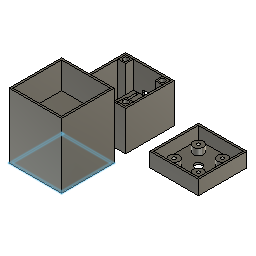
TeamsStatusLight (Autodesk Fusion 360 design; units mm, degrees)
Autodesk Fusion 360 part; units mm, degrees
sketch "Sketch1" plane through (0, 0, 0) normal (0, 0, 1) x (1, 0, 0)
  line L0 (1.4665, 38.7145) -> (39.4665, 38.7145)
  line L1 (39.4665, 38.7145) -> (39.4665, 0.7145)
  line L2 (39.4665, 0.7145) -> (1.4665, 0.7145)
  line L3 (1.4665, 0.7145) -> (1.4665, 38.7145)
  dimension "d4" = 38
  dimension "d5" = 38
  constraint horizontal L0
  constraint vertical L1
  constraint horizontal L2
  constraint vertical L3
  measures "d4" distance of L0.start L0.end
  measures "d5" distance of L0.start L2.end
extrude "Extrude1" add sketch "Sketch1" along normal blind 1.5 makes body 1
sketch "Sketch2" plane through (0, 0, 1.5) normal (0, 0, 1) x (-1, 0, 0)
  line L0 (-1.4665, -0.7145) -> (-39.4665, -0.7145)
  line L1 (-39.4665, -0.7145) -> (-39.4665, -38.7145)
  line L2 (-39.4665, -38.7145) -> (-1.4665, -38.7145)
  line L3 (-1.4665, -38.7145) -> (-1.4665, -0.7145)
  line L4 (-1.4665, -38.7145) -> (-2.9665, -38.7145)
  line L5 (-2.9665, -38.7145) -> (-2.9665, -37.2145)
  line L6 (-2.9665, -37.2145) -> (-37.9665, -37.2145)
  line L7 (-37.9665, -37.2145) -> (-37.9665, -2.2145)
  line L8 (-37.9665, -2.2145) -> (-2.9665, -2.2145)
  line L9 (-2.9665, -2.2145) -> (-2.9665, -37.2145)
  dimension "d8" = 1.5
  dimension "d9" = 1.5
  dimension "d10" = 35
  dimension "d11" = 35
  constraint coincident L2.end L3.start
  constraint perpendicular L3 L4
  constraint perpendicular L2 L5
  constraint horizontal L6
  constraint vertical L7
  constraint horizontal L8
  constraint vertical L9
  measures "d8" distance of L2.end L4.end
  measures "d9" distance of L4.end L5.end
  measures "d10" distance of L5.end L6.end
  measures "d11" distance of L5.end L8.end
extrude "Extrude2" add sketch "Sketch2" along normal blind 40 bodies 1
ref_plane "WorkPlane1" through (20.4665, 19.7145, 20.75) normal (0, 1, 0) x (-1, 0, 0)
ref_plane "WorkPlane2" through (20.4665, 19.7145, 20.75) normal (-1, 0, 0) x (0, -1, 0)
sketch "Sketch3" plane through (0, 38.7145, 0) normal (0, 1, 0) x (-1, 0, 0)
  line L0 (-39.4665, 0) -> (-1.4665, 0)
  line L1 (-1.4665, 0) -> (-1.4665, 41.5)
  line L2 (-1.4665, 41.5) -> (-39.4665, 41.5)
  line L3 (-39.4665, 41.5) -> (-39.4665, 0)
  line L4 (-20.4665, 0) -> (-20.4665, 1.5)
  line L5 (-20.4665, 1.5) -> (-20.4665, 12)
  line L6 (-16.9665, 13.75) -> (-23.9665, 13.75)
  line L7 (-24.9665, 12.75) -> (-24.9665, 11.25)
  line L8 (-23.9665, 10.25) -> (-16.9665, 10.25)
  line L9 (-15.9665, 11.25) -> (-15.9665, 12.75)
  line L10 (-15.9665, 13.75) -> (-24.9665, 10.25) construction
  line L11 (-24.9665, 13.75) -> (-15.9665, 10.25) construction
  arc A0 (-23.9665, 13.75) -> (-24.9665, 12.75) centre (-23.9665, 12.75) ccw
  arc A1 (-24.9665, 11.25) -> (-23.9665, 10.25) centre (-23.9665, 11.25) ccw
  arc A2 (-16.9665, 10.25) -> (-15.9665, 11.25) centre (-16.9665, 11.25) ccw
  arc A3 (-15.9665, 12.75) -> (-16.9665, 13.75) centre (-16.9665, 12.75) ccw
  point P0 (-20.4665, 12)
  dimension "d18" = 1.5
  dimension "d19" = 10.5
  dimension "d20" = 9
  dimension "d21" = 3.5
  dimension "d22" = 1
  constraint midpoint L0 L4.start
  constraint perpendicular L0 L4
  constraint parallel L4 L5
  constraint horizontal L6
  constraint perpendicular L6 L7
  constraint parallel L6 L8
  constraint parallel L7 L9
  constraint coincident L10 P0
  constraint coincident L11 P0
  constraint coincident P0 L5.end
  constraint coincident L11.start L6
  constraint coincident L11.start L7
  constraint tangent L6 A0
  constraint tangent L7 A0
  constraint coincident L10.end L7
  constraint coincident L10.end L8
  constraint tangent L7 A1
  constraint tangent L8 A1
  constraint equal A0 A1
  constraint coincident L11.end L9
  constraint coincident L11.end L8
  constraint tangent L9 A2
  constraint tangent L8 A2
  constraint equal A0 A2
  constraint coincident L10.start L9
  constraint coincident L10.start L6
  constraint tangent L9 A3
  constraint tangent L6 A3
  constraint equal A0 A3
  measures "d18" distance of L4.start L4.end
  measures "d19" distance of L4.end P0
  measures "d20" distance of L10.end L11.end
  measures "d21" distance of L11.start L10.end
  measures "d22" radius of A0
extrude "Extrude3" cut sketch "Sketch3" against normal blind 1.5 contours L6 L7 L8 L9 A0 A1 A2 A3 bodies 1
sketch "Sketch4" plane through (0, 0, 1.5) normal (0, 0, 1) x (-1, 0, 0)
  line L0 (-37.9665, -2.2145) -> (-37.9665, -37.2145)
  line L1 (-37.9665, -37.2145) -> (-2.9665, -37.2145)
  line L2 (-2.9665, -37.2145) -> (-2.9665, -2.2145)
  line L3 (-2.9665, -2.2145) -> (-37.9665, -2.2145)
  line L4 (-20.4665, -37.2145) -> (-20.4665, -25.4645)
  line L5 (-11.3165, -37.2145) -> (-29.6165, -37.2145)
  line L6 (-29.6165, -37.2145) -> (-29.6165, -13.7145)
  line L7 (-29.6165, -13.7145) -> (-11.3165, -13.7145)
  line L8 (-11.3165, -13.7145) -> (-11.3165, -37.2145)
  line L9 (-11.3165, -37.2145) -> (-29.6165, -13.7145) construction
  line L10 (-29.6165, -37.2145) -> (-11.3165, -13.7145) construction
  point P0 (-20.4665, -25.4645)
  dimension "d29" = 11.75
  dimension "d30" = 18.3
  dimension "d31" = 23.5
  constraint midpoint L1 L4.start
  constraint perpendicular L1 L4
  constraint horizontal L5
  constraint perpendicular L5 L6
  constraint parallel L5 L7
  constraint parallel L6 L8
  constraint coincident L9 P0
  constraint coincident L10 P0
  constraint coincident P0 L4.end
  measures "d29" distance of L4.start P0
  measures "d30" distance of L6.end L7.end
  measures "d31" distance of L5.end L6.end
extrude "Extrude4" add sketch "Sketch4" along normal blind 8.5 contours L1 L5 L6 L7 L8 bodies 1
sketch "Sketch5" plane through (0, 0, 10) normal (0, 0, 1) x (-1, 0, 0)
  line L0 (-11.3165, -13.7145) -> (-29.6165, -13.7145)
  line L1 (-29.6165, -13.7145) -> (-29.6165, -37.2145)
  line L2 (-29.6165, -37.2145) -> (-11.3165, -37.2145)
  line L3 (-11.3165, -37.2145) -> (-11.3165, -13.7145)
  line L4 (-29.6165, -13.7145) -> (-25.6165, -13.7145)
  line L5 (-25.6165, -13.7145) -> (-25.6165, -15.2145)
  point P0 (-22.9498, -15.2145)
  point P1 (-20.2831, -15.2145)
  point P2 (-17.6165, -15.2145)
  dimension "d34" = 4
  dimension "d35" = 1.5
  dimension "d38" = 8
  dimension "d39" = 0
  constraint coincident L0.end L1.start
  constraint perpendicular L1 L4
  constraint perpendicular L4 L5
  measures "d34" distance of L0.end L4.end
  measures "d35" distance of L4.end L5.end
hole "Hole1" at (25.6165, 15.2145, 10) at (22.9498, 15.2145, 10) at (20.2831, 15.2145, 10) at (17.6165, 15.2145, 10) direction (0, 0, -1) diameter 0.7 depth 7 tip angle 180 bodies 1
ref_plane "WorkPlane3" through (20.4665, 19.7145, 20.75) normal (0, 0, 1) x (1, 0, 0)
split "Split1" by plane through (20.4665, 19.7145, 20.75) normal (0, 0, 1) bodies 1 makes body 2 at (1.4665, 13.3812, 27.6667)
move_body "Move1" bodies 2 to x (1, 0, 0) y (0, 1, 0) z (0, 0, 1) at (57, 0, 0)
ref_plane "WorkPlane4" through (77.4665, 19.7145, 31.125) normal (1, 0, 0) x (0, 1, 0)
ref_plane "WorkPlane5" through (77.4665, 19.7145, 31.125) normal (0, 1, 0) x (-1, 0, 0)
sketch "Sketch6" plane through (0, 37.2145, 0) normal (0, -1, 0) x (1, 0, 0)
  line L0 (59.9665, 20.75) -> (94.9665, 20.75)
  line L1 (94.9665, 20.75) -> (94.9665, 41.5)
  line L2 (94.9665, 41.5) -> (59.9665, 41.5)
  line L3 (59.9665, 41.5) -> (59.9665, 20.75)
  line L4 (59.9665, 20.75) -> (94.9665, 20.75)
  line L5 (94.9665, 20.75) -> (94.9665, 22.25)
  line L6 (94.9665, 22.25) -> (59.9665, 22.25)
  line L7 (59.9665, 22.25) -> (59.9665, 20.75)
  dimension "d43" = 35
  dimension "d44" = 1.5
  constraint horizontal L4
  constraint vertical L5
  constraint horizontal L6
  constraint vertical L7
  constraint coincident L0.start L3.end
  measures "d43" distance of L0.start L0.end
  measures "d44" distance of L0.start L6.end
extrude "Extrude5" add sketch "Sketch6" along normal blind 35 contours L0 L1 L3 L4 L5 L6 L7 bodies 2
sketch "Sketch7" plane through (0, 0, 22.25) normal (0, 0, 1) x (-1, 0, 0)
  line L0 (-94.9665, -37.2145) -> (-59.9665, -37.2145)
  line L1 (-59.9665, -37.2145) -> (-59.9665, -2.2145)
  line L2 (-59.9665, -2.2145) -> (-94.9665, -2.2145)
  line L3 (-94.9665, -2.2145) -> (-94.9665, -37.2145)
  line L4 (-59.9665, -37.2145) -> (-67.9665, -37.2145)
  line L5 (-67.9665, -37.2145) -> (-67.9665, -29.2145)
  circle A0 centre (-67.9665, -29.2145) radius 4
  line L6 (-100.2665, -19.7145) -> (-54.6665, -19.7145)
  circle A1 centre (-67.9665, -10.2145) radius 4
  line L7 (-77.4665, 3.0855) -> (-77.4665, -42.5145)
  circle A2 centre (-86.9665, -29.2145) radius 4
  circle A3 centre (-86.9665, -10.2145) radius 4
  dimension "d47" = 8
  dimension "d50" = 8
  dimension "d51" = 8
  constraint coincident L0.end L1.start
  constraint perpendicular L1 L4
  constraint perpendicular L0 L5
  constraint coincident L5.end A0.centre
  constraint symmetric A0 L6 A1
  constraint symmetric A0 L7 A2
  constraint symmetric A1 L7 A3
  measures "d47" distance of L0.end L4.end
  measures "d50" distance of L4.end L5.end
  measures "d51" diameter of A0
extrude "Extrude6" add sketch "Sketch7" along normal blind 5 contours A0 | A1 | A2 | A3 bodies 2
hole "Hole3" at (67.9665, 29.2145, 27.25) direction (0, 0, -1) diameter 2.529 depth 4 tip angle 180 bodies 2
thread "Thread2" "ISO Metric profile 3.0 M3x0.5 6H" thread offset 0 thread depth 7.4
mirror "Mirror1" about plane through (77.4665, 19.7145, 31.125) normal (1, 0, 0) of "Hole3"
mirror "Mirror2" about plane through (77.4665, 19.7145, 31.125) normal (0, 1, 0) of "Hole3", "Mirror1"
hole "Hole4" at (77.4665, 19.7145, 22.25) direction (0, 0, -1) diameter 6 depth 4 tip angle 180 bodies 2
sketch "Sketch9" plane through (0, 0, 1.5) normal (0, 0, 1) x (-1, 0, 0)
  line L0 (-29.6165, -37.2145) -> (-29.6165, -13.7145)
  line L1 (-29.6165, -13.7145) -> (-11.3165, -13.7145)
  line L2 (-11.3165, -13.7145) -> (-11.3165, -37.2145)
  line L3 (-11.3165, -37.2145) -> (-2.9665, -37.2145)
  line L4 (-2.9665, -37.2145) -> (-2.9665, -2.2145)
  line L5 (-2.9665, -2.2145) -> (-37.9665, -2.2145)
  line L6 (-37.9665, -2.2145) -> (-37.9665, -37.2145)
  line L7 (-37.9665, -37.2145) -> (-29.6165, -37.2145)
  line L8 (-2.9665, -37.2145) -> (-8.9665, -37.2145)
  line L9 (-8.9665, -37.2145) -> (-8.9665, -31.2145)
  line L10 (-8.9665, -31.2145) -> (-2.9665, -31.2145)
  line L11 (-2.9665, -31.2145) -> (-2.9665, -37.2145)
  line L12 (-43.2665, -19.7145) -> (2.3335, -19.7145)
  line L13 (-2.9665, -2.2145) -> (-8.9665, -2.2145)
  line L14 (-8.9665, -2.2145) -> (-8.9665, -8.2145)
  line L15 (-8.9665, -8.2145) -> (-2.9665, -8.2145)
  line L16 (-2.9665, -8.2145) -> (-2.9665, -2.2145)
  line L17 (-20.4665, -42.5145) -> (-20.4665, 3.0855)
  line L18 (-31.9665, -31.2145) -> (-37.9665, -31.2145)
  line L19 (-37.9665, -31.2145) -> (-37.9665, -37.2145)
  line L20 (-37.9665, -37.2145) -> (-31.9665, -37.2145)
  line L21 (-31.9665, -37.2145) -> (-31.9665, -31.2145)
  line L22 (-31.9665, -8.2145) -> (-37.9665, -8.2145)
  line L23 (-37.9665, -8.2145) -> (-37.9665, -2.2145)
  line L24 (-31.9665, -2.2145) -> (-31.9665, -8.2145)
  line L25 (-37.9665, -2.2145) -> (-31.9665, -2.2145)
  dimension "d75" = 6
  dimension "d76" = 6
  constraint horizontal L8
  constraint vertical L9
  constraint horizontal L10
  constraint vertical L11
  constraint coincident L3.end L4.start
  constraint symmetric L3.end L12 L4.end
  constraint symmetric L8.end L12 L13.end
  constraint symmetric L9.end L12 L14.end
  constraint symmetric L10.end L12 L15.end
  constraint symmetric L3.end L17 L6.end
  constraint symmetric L8.end L17 L20.end
  constraint symmetric L9.end L17 L18.start
  constraint symmetric L10.end L17 L18.end
  constraint symmetric L4.end L17 L5.end
  constraint symmetric L13.end L17 L24.start
  constraint symmetric L14.end L17 L22.start
  constraint symmetric L15.end L17 L22.end
  measures "d75" distance of L3.end L8.end
  measures "d76" distance of L3.end L10.end
extrude "Extrude7" add sketch "Sketch9" along normal blind 19 contours L6 L7 L18 L19 L20 L21 | L5 L6 L22 L23 L24 L25 | L4 L5 L13 L14 L15 L16 | L3 L4 L8 L9 L10 L11 bodies 1
hole "Hole5" at (34.9665, 5.2145, 20.5) direction (0, 0, -1) diameter 4.1 depth 6 tip angle 180 bodies 1
mirror "Mirror3" about plane through (20.4665, 19.7145, 20.75) normal (-1, 0, 0) of "Hole5"
mirror "Mirror4" about plane through (20.4665, 19.7145, 20.75) normal (0, 1, 0) of "Hole5", "Mirror3"
sketch "Sketch8" plane through (0, 0, 22.25) normal (0, 0, 1) x (-1, 0, 0)
  circle A0 centre (-77.4665, -19.7145) radius 3
  circle A1 centre (-67.9665, -10.2145) radius 4
  circle A2 centre (-67.9665, -29.2145) radius 4
  circle A3 centre (-86.9665, -10.2145) radius 4
  circle A4 centre (-86.9665, -29.2145) radius 4
  line L0 (-94.9665, -37.2145) -> (-59.9665, -37.2145)
  line L1 (-59.9665, -37.2145) -> (-59.9665, -2.2145)
  line L2 (-59.9665, -2.2145) -> (-94.9665, -2.2145)
  line L3 (-94.9665, -2.2145) -> (-94.9665, -37.2145)
  line L4 (-59.9665, -37.2145) -> (-62.9665, -37.2145)
  line L5 (-62.9665, -37.2145) -> (-62.9665, -34.2145)
  line L6 (-77.4665, 3.0855) -> (-77.4665, -42.5145)
  line L7 (-100.2665, -19.7145) -> (-54.6665, -19.7145)
  point P0 (-91.9665, -34.2145)
  point P1 (-62.9665, -5.2145)
  point P2 (-91.9665, -5.2145)
  dimension "d86" = 3
  dimension "d87" = 3
  constraint coincident L0.end L1.start
  constraint perpendicular L1 L4
  constraint perpendicular L0 L5
  constraint symmetric L5.end L6 P0
  constraint symmetric L5.end L7 P1
  constraint symmetric P0 L7 P2
  measures "d86" distance of L0.end L4.end
  measures "d87" distance of L4.end L5.end
hole "Hole6" at (62.9665, 34.2145, 22.25) at (91.9665, 34.2145, 22.25) at (91.9665, 5.2145, 22.25) at (62.9665, 5.2145, 22.25) direction (0, 0, -1) diameter 3.1 depth 1.5 tip angle 180 bodies 2
move_body "Move2" bodies 2 to x (1, 0, 0) y (0, 1, 0) z (0, 0, 1) at (0, 0, -20.7)
sketch "Sketch10" plane through (0, 0, 0) normal (0, 0, 1) x (1, 0, 0)
  line L0 (0, -10) -> (41.15, -10)
  line L1 (41.15, -10) -> (41.15, -51.15)
  line L2 (41.15, -51.15) -> (0, -51.15)
  line L3 (0, -51.15) -> (0, -10)
  line L4 (0, -10) -> (1.5, -10)
  line L5 (1.5, -10) -> (1.5, -11.5)
  line L6 (1.5, -11.5) -> (39.65, -11.5)
  line L7 (39.65, -11.5) -> (39.65, -49.65)
  line L8 (39.65, -49.65) -> (1.5, -49.65)
  line L9 (1.5, -49.65) -> (1.5, -11.5)
  dimension "d91" = 41.15
  dimension "d92" = 41.15
  dimension "d93" = 1.5
  dimension "d94" = 1.5
  dimension "d95" = 38.15
  dimension "d96" = 38.15
  constraint horizontal L0
  constraint vertical L1
  constraint horizontal L2
  constraint vertical L3
  constraint perpendicular L3 L4
  constraint perpendicular L0 L5
  constraint horizontal L6
  constraint vertical L7
  constraint horizontal L8
  constraint vertical L9
  measures "d91" distance of L0.start L0.end
  measures "d92" distance of L0.start L2.end
  measures "d93" distance of L0.start L4.end
  measures "d94" distance of L4.end L5.end
  measures "d95" distance of L5.end L6.end
  measures "d96" distance of L5.end L8.end
extrude "Extrude8" add sketch "Sketch10" along normal blind 30 separate body contours L6 L7 L8 L9 makes body 3
extrude "Extrude9" add sketch "Sketch10" along normal blind 50.8 bodies 3
extrude "Extrude10" cut 1 faces at (83.2998, 1.2145, 20.8) along direction (0, 0, -1) blind 9.5 on bodies 2 bodies 2
extrude "Extrude11" add 1 faces at (14.6331, 1.2145, 20.75) along direction (0, 0, 1) blind 10 on bodies 1 bodies 1
extrude "Extrude12" add 4 faces at (37.6479, 34.1634, 20.5) (32.285, 5.2656, 20.5) (8.6479, 5.1634, 20.5) (8.6479, 34.1634, 20.5) along direction (0, 0, 1) blind 10.3 on bodies 1 bodies 1
extrude "Extrude13" add 1 faces at (17.4165, 13.7145, 7.1667) along direction (0, -1, 0) blind 3 on bodies 1 bodies 1
sketch "Sketch11" plane through (0, 0, 10) normal (0, 0, 1) x (-1, 0, 0)
  circle A0 centre (-20.2831, -15.2145) radius 0.35
  circle A1 centre (-25.6165, -15.2145) radius 0.35
  circle A2 centre (-22.9498, -15.2145) radius 0.35
  circle A3 centre (-17.6165, -15.2145) radius 0.35
  line L0 (-29.6165, -10.7145) -> (-29.6165, -37.2145)
  line L1 (-29.6165, -37.2145) -> (-11.3165, -37.2145)
  line L2 (-11.3165, -37.2145) -> (-11.3165, -10.7145)
  line L3 (-11.3165, -10.7145) -> (-29.6165, -10.7145)
  line L4 (-29.6165, -15.0777) -> (-27.9165, -15.0777)
  line L5 (-11.3165, -15.0347) -> (-13.0165, -15.0347)
  line L6 (-28.7665, -15.0777) -> (-27.0665, -15.0777)
  line L7 (-27.0665, -15.0777) -> (-27.0665, -36.8777)
  line L8 (-27.0665, -36.8777) -> (-28.7665, -36.8777)
  line L9 (-28.7665, -36.8777) -> (-28.7665, -15.0777)
  line L10 (-20.4665, -42.5145) -> (-20.4665, 3.0855)
  line L11 (-13.8665, -15.0777) -> (-13.8665, -36.8777)
  line L12 (-12.1665, -36.8777) -> (-12.1665, -15.0777)
  line L13 (-12.1665, -15.0777) -> (-13.8665, -15.0777)
  line L14 (-13.8665, -36.8777) -> (-12.1665, -36.8777)
  line L15 (-27.9165, -15.0777) -> (-27.9165, -15.9277)
  line L16 (-27.9165, -15.9277) -> (-13.0165, -15.9277)
  line L17 (-13.0165, -15.9277) -> (-13.0165, -14.2277)
  line L18 (-13.0165, -14.2277) -> (-27.9165, -14.2277)
  line L19 (-27.9165, -14.2277) -> (-27.9165, -15.9277)
  dimension "d109" = 1.7
  dimension "d110" = 1.7
  dimension "d115" = 1.7
  dimension "d116" = 21.8
  dimension "d117" = 0.85
  dimension "d118" = 14.9
  dimension "d119" = 1.7
  constraint coincident L0 L4.start
  constraint perpendicular L0 L4
  constraint coincident L2 L5.start
  constraint perpendicular L2 L5
  constraint horizontal L6
  constraint vertical L7
  constraint horizontal L8
  constraint vertical L9
  constraint midpoint L4 L6.start
  constraint symmetric L6.start L10 L12.end
  constraint symmetric L6.end L10 L11.start
  constraint symmetric L7.end L10 L11.end
  constraint symmetric L8.end L10 L12.start
  constraint perpendicular L6 L15
  constraint horizontal L16
  constraint vertical L17
  constraint horizontal L18
  constraint vertical L19
  measures "d109" distance of L4.start L4.end
  measures "d110" distance of L5.start L5.end
  measures "d115" distance of L6.start L6.end
  measures "d116" distance of L6.start L8.end
  measures "d117" distance of L4.end L15.end
  measures "d118" distance of L15.end L16.end
  measures "d119" distance of L15.end L18.end
extrude "Extrude14" add 1 faces at (29.6165, 28.3812, 4.3333) along direction (1, 0, 0) blind 2 on bodies 1 bodies 1
extrude "Extrude15" add 1 faces at (11.3165, 19.5478, 4.3333) along direction (-1, 0, 0) blind 2 on bodies 1 bodies 1
extrude "Extrude16" cut sketch "Sketch11" against normal blind 6.5 contours A0 L10 L11 L13 L16 L17 L18 | A0 L6 L7 L10 L16 L18 L19 | L6 L7 L15 L16 L19 | L4 L6 L7 L8 L9 L15 L16 L19 | L11 L12 L13 L14 L16 L17 | L11 L13 L16 L17 bodies 1
equation "matrix_pcb_w = 35 mm"
equation "matrix_pcb_l = 35 mm"
equation "wall_thick = 1.5 mm"
equation "d4 = matrix_pcb_w + wall_thick * 2"
equation "d5 = matrix_pcb_l + wall_thick * 2"
equation "d6 = wall_thick"
equation "d8 = wall_thick"
equation "d9 = wall_thick"
equation "d10 = matrix_pcb_w"
equation "d11 = matrix_pcb_l"
equation "pin_height = 6 mm"
equation "pin_pitch = 2 mm"
equation "usb_width = 9 mm"
equation "usb_height = 3.5 mm"
equation "d18 = wall_thick"
equation "d19 = pin_height + usb_height + 1 mm"
equation "d20 = usb_width"
equation "d21 = usb_height"
equation "d23 = -wall_thick"
equation "rpi_width = 18.3 mm"
equation "rpi_len = 23.5 mm"
equation "rpi_pin_inset = 1.5 mm"
equation "pin_width = 0.7 mm"
equation "d29 = rpi_len / 2"
equation "d30 = rpi_width"
equation "d31 = rpi_len"
equation "d32 = pin_height + usb_height - 1 mm"
equation "d35 = rpi_pin_inset"
equation "d38 = 4 * pin_pitch"
equation "d40 = pin_height + 1 mm"
equation "d41 = pin_width"
equation "d43 = matrix_pcb_w"
equation "d44 = wall_thick"
equation "d45 = matrix_pcb_l"
equation "d47 = matrix_hole_x"
equation "matrix_hole_x = 8 mm"
equation "matrix_hole_y = 8 mm"
equation "d50 = matrix_hole_y"
equation "d51 = matrix_hole_x"
equation "d88 = wall_thick"
equation "d91 = matrix_pcb_w + 4 * wall_thick + 0.15 mm"
equation "d92 = matrix_pcb_w + 4 * wall_thick + 0.15 mm"
equation "d93 = wall_thick"
equation "d94 = wall_thick"
equation "d95 = matrix_pcb_w + 2 * wall_thick + 0.15 mm"
equation "d96 = matrix_pcb_w + 2 * wall_thick + 0.15 mm"
equation "d116 = rpi_len - 1.7 mm"
equation "d118 = rpi_width - ( 1.7 * 2 ) * 1 mm"
named bodies: "rpi_2040_zero_bottom", "Matrix_holder", "clear-light-path"
